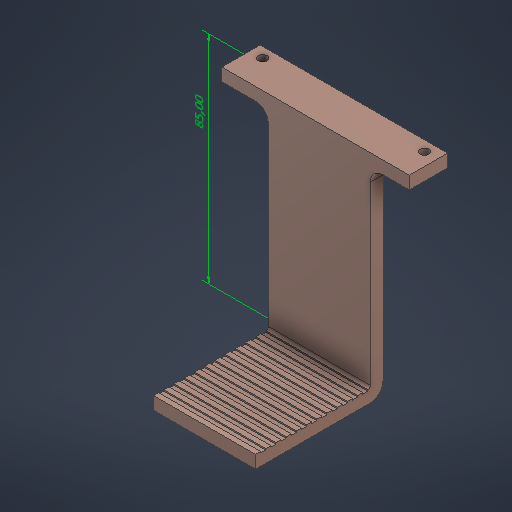
# Autodesk Inventor part: Garra inferior
Saved by Autodesk Inventor 2026 (Build 300175000, 175)
## iProperties
Created: 2025-08-24
Part Number: Garra inferior
Material: Plástico PC/ABS
Document SubType Name: Modeling
Designer: Thomas
Density: 1.1 g/cm^3
Appearance: Suave - Blanco
Author: Thomas
Autodesk Inventor part; units mm, degrees
ref_plane "YZ Plane" through (0, 0, 0) normal (1, 0, 0) x (0, 1, 0)
ref_plane "XZ Plane" through (0, 0, 0) normal (0, 1, 0) x (-1, 0, 0)
ref_plane "XY Plane" through (0, 0, 0) normal (0, 0, 1) x (1, 0, 0)
sketch "Boceto1" plane through (0, 0, 0) normal (1, 0, 0) x (0, 1, 0)
  line L0 (0, 0) -> (80, 0)
  line L1 (0, 0) -> (0, 50)
  line L2 (80, 0) -> (80, -10)
  line L3 (85, -10) -> (85, 5)
  line L4 (85, 5) -> (5, 5)
  line L5 (5, 5) -> (5, 50)
  line L6 (80, -10) -> (85, -10)
  line L7 (0, 50) -> (5, 50)
  dimension "d0" = 80
  dimension "d1" = 50
  dimension "d2" = 10
  dimension "d3" = 5
  constraints: 16 end point, 3 horizontal, 2 vertical, 2 other
  measures "d0" distance of L0.start L0.end
  measures "d1" distance of L0.start L1.end
  measures "d2" distance of L0.end L2.end
  measures "d3" distance between parallel lines of L2 L3
extrude "Extrusión1" add sketch "Boceto1" along normal mid plane 73.5
sketch "Boceto2" plane through (-36.75, 5, 50) normal (0, 1, 0) x (1, 0, 0)
  line L0 (0, 45) -> (73.5, 45) projected
  line L1 (18.2, 45) -> (18.2, 0)
  line L2 (0, 0) -> (73.5, 0) projected
  line L3 (58.2, 58.7474) -> (58.2, 0)
  line L4 (0, 0) -> (0, 45) projected
  line L5 (73.5, 45) -> (73.5, 0) projected
  point P0 (36.75, 50)
  point P1 (36.75, 0)
  point P2 (58.2, 45)
  point P3 (58.2, 0)
  dimension "d6" = 40
  dimension "d7" = 18.55
  constraints: 4 end point, 2 point on line, 2 vertical, 1 midpoint
  measures "d6" distance between parallel lines of L3 L1
  measures "d7" distance from line of L1 point (36.75, 0)
extrude "Extrusión2" cut sketch "Boceto2" against normal through all contours L0 L1 L2 L4 | L0 L5 L2 L3
sketch "Boceto3" plane through (-36.75, 85, 5) normal (0, 0, 1) x (1, 0, 0)
  line L0 (0, -5) -> (73.5, -5) projected
  line L1 (18.2, -80) -> (18.2, -85) projected
  line L2 (0, -5) -> (18.2, -5)
  line L3 (18.2, -5) -> (18.2, -85)
  line L4 (18.2, -85) -> (0, -85)
  line L5 (0, -85) -> (0, -5)
  line L6 (58.2, -80) -> (58.2, -85) projected
  line L7 (58.2, -85) -> (73.5, -85)
  line L8 (73.5, -85) -> (73.5, -5)
  line L9 (73.5, -5) -> (58.2, -5)
  line L10 (58.2, -5) -> (58.2, -85)
  point P0 (36.75, -85)
  point P1 (58.2, -5)
  constraints: 16 end point, 4 parallel, 2 horizontal, 2 perpendicular, 1 point on line
extrude "Extrusión3" cut sketch "Boceto3" against normal through all
fillet "Empalme1" radius 5 1 edges at (1.45, 80, 0)
fillet "Empalme2" radius 5 1 edges at (1.45, 0, 0)
sketch "Boceto4" plane through (-36.75, 80, -10) normal (0, -1, 0) x (1, 0, 0)
  circle A0 centre (5, 4) radius 1.75
  circle A1 centre (5, 4) radius 3 construction
  line L0 (0, 0) -> (73.5, 0) projected
  line L1 (0, 0) -> (0, 10) projected
  point P0 (36.75, 10)
  point P1 (0, 15)
  dimension "d14" = 3.5
  dimension "d15" = 6
  dimension "d16" = 4
  dimension "d17" = 5
  constraints: 2 centre point, 1 coincident
  measures "d14" diameter of A0
  measures "d15" diameter of A1
  measures "d16" distance from line of A0.centre L0
  measures "d17" distance from line of L1 A0.centre
extrude "Extrusión4" cut sketch "Boceto4" against normal through all
mirror "Simetría1" about plane through (0, 0, 0) normal (1, 0, 0) of "Extrusión4"
fillet "Empalme3" radius 1 1 edges at (1.45, 5, 5)
sketch "Boceto5" plane through (21.45, 0, 50) normal (1, 0, 0) x (0, 0, -1)
  line L0 (0, 5) -> (44, 5) projected
  line L1 (0, 5) -> (2, 5)
  line L2 (2, 5) -> (2, 4.5)
  line L3 (2, 4.5) -> (4, 4.5)
  line L4 (4, 4.5) -> (4, 5)
  line L5 (0, 0) -> (0, 5) projected
  point P0 (50, 0)
  dimension "d21" = 2
  dimension "d22" = 2
  dimension "d23" = 0.5
  constraints: 8 end point, 2 perpendicular, 2 point on line, 1 vertical
  measures "d21" distance between parallel lines of L5 L2
  measures "d22" distance of L2.end L3.end
  measures "d23" distance of L1.end L2.end
extrude "Extrusión5" cut sketch "Boceto5" against normal through all
pattern_linear "Patrón rectangular1" count 11 spacing 4 along (0, 0, -1) of "Extrusión5"
fillet "Empalme4" radius 5 2 edges at (-18.55, 80, 0) (21.45, 80, 0)
sketch "Boceto6" plane through (0, 0, 0) normal (1, 0, 0) x (0, 1, 0)
  arc A0 (0, 5) -> (5, 0) centre (5, 5) ccw construction
  line L0 (80, 5) -> (80, -10) construction
  line L1 (5, 0) -> (80, -10)
  point P0 (0, 0)
  constraints: 2 end point
extrude "Nervio1" add sketch "Boceto6" along normal mid plane 8 rib yes fills toward (42.5066, -4.9504) open curves L1
equation "\"d22\" = d21"
